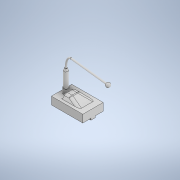
# Autodesk Inventor part: 準確無線麥克風組
Saved by Autodesk Inventor 2021 (Build 250183000, 183)
## iProperties
Created: 2023-02-28
Part Number: 準確無線麥克風組
Material: 一般
Document SubType Name: Modeling
Designer: brian
Density: 1 g/cm^3
Appearance: 預設
Author: brian
Autodesk Inventor part; units mm, degrees
ref_plane "YZ Plane" through (0, 0, 0) normal (1, 0, 0) x (0, 1, 0)
ref_plane "XZ Plane" through (0, 0, 0) normal (0, 1, 0) x (-1, 0, 0)
sketch "草圖1" plane through (0, 0, 0) normal (0, 1, 0) x (-1, 0, 0)
  line L0 (76.2, 49.6) -> (-76.2, 49.6)
  line L1 (-76.2, 49.6) -> (-76.2, -49.6)
  line L2 (-76.2, -49.6) -> (76.2, -49.6)
  line L3 (76.2, -49.6) -> (76.2, 49.6)
  line L4 (76.2, 49.6) -> (-76.2, -49.6) construction
  line L5 (-76.2, 49.6) -> (76.2, -49.6) construction
  point P0 (0, 0)
  dimension "d0" = 152.4
  dimension "d1" = 99.2
  constraints: 12 end point, 2 midpoint, 2 parallel, 1 horizontal, 1 perpendicular
  measures "d0" distance of L2.end L1.end
  measures "d1" distance of L1.end L0.end
extrude "擠出1" add sketch "草圖1" along normal blind 37
sketch "草圖2" plane through (0, 0, 0) normal (0, -1, 0) x (1, 0, 0)
  line L0 (76.2, 49.6) -> (76.2, -49.6) projected
  line L1 (65.2, 10) -> (76.2, 10)
  line L2 (76.2, 10) -> (76.2, -10)
  line L3 (76.2, -10) -> (65.2, -10)
  line L4 (65.2, -10) -> (65.2, 10)
  point P0 (0, 0)
  point P1 (65.2, 0)
  point P2 (76.2, 0)
  dimension "d4" = 20
  dimension "d5" = 11
  constraints: 8 end point, 2 midpoint, 2 parallel, 1 horizontal, 1 horizontal alignment, 1 perpendicular, 1 point on line
  measures "d4" distance of L3.end L1.start
  measures "d5" distance between parallel lines of L0 L4
extrude "擠出2" add sketch "草圖2" along normal blind 8
sketch "草圖3" plane through (0, 37, 0) normal (0, 1, 0) x (1, 0, 0)
  line L0 (-42.2, -36) -> (47.8, -36)
  line L1 (47.8, -36) -> (47.8, 36)
  line L2 (47.8, 36) -> (-42.2, 36)
  line L3 (-42.2, 36) -> (-42.2, -36)
  line L4 (-42.2, -36) -> (47.8, 36) construction
  line L5 (47.8, -36) -> (-42.2, 36) construction
  line L6 (-76.2, 49.6) -> (-76.2, -49.6) projected
  point P0 (2.8, 0)
  dimension "d8" = 90
  dimension "d9" = 72
  dimension "d14" = 34
  constraints: 12 end point, 2 midpoint, 2 parallel, 1 horizontal, 1 perpendicular
  measures "d8" distance of L2.end L1.end
  measures "d9" distance of L1.end L0.end
  measures "d14" distance between parallel lines of L6 L3
extrude "擠出3" add sketch "草圖3" along normal blind 16
sketch "草圖4" plane through (0, 37, 0) normal (0, 1, 0) x (1, 0, 0)
  circle A0 centre (-55.2, 0) radius 12.5
  line L0 (-76.2, 49.6) -> (-76.2, -49.6) projected
  point P0 (0, 0)
  point P1 (-76.2, 0)
  dimension "d12" = 25
  dimension "d13" = 21
  constraints: 1 centre point, 1 horizontal alignment, 1 midpoint
  measures "d12" diameter of A0
  measures "d13" distance from line of L0 A0.centre
extrude "擠出4" add sketch "草圖4" along normal blind 22
sketch "草圖5" plane through (-55.2, 59, 0) normal (0, 1, 0) x (1, 0, 0)
  circle A0 centre (0, 0) radius 12.5 projected
  circle A1 centre (0, 0) radius 10
  point P0 (55.2, 0)
  dimension "d17" = 20
  constraints: 1 centre point, 1 coincident
  measures "d17" diameter of A1
extrude "擠出5" add sketch "草圖5" along normal blind 72 contours A1
ref_plane "工作平面1" through (-55.2, 141, 0) normal (0, 1, 0) x (1, 0, 0)
sketch "草圖6" plane through (-55.2, 141, 0) normal (0, 1, 0) x (1, 0, 0)
  circle A0 centre (0, 0) radius 10 construction
  circle A1 centre (0, 0) radius 6.25
  point P0 (55.2, 0)
  dimension "d21" = 12.5
  constraints: 1 centre point, 1 coincident
  measures "d21" diameter of A1
loft "斷面混成1" add profiles "草圖6" section 1 edges at (-65.2, 131, 0)
sketch "草圖7" plane through (-55.2, 141, 0) normal (0, 1, 0) x (1, 0, 0)
  circle A0 centre (0, 0) radius 6.25 projected
  line L0 (0, 0) -> (147.496, -68.7785)
  line L1 (0, 0) -> (162.7438, 0) construction
  point P0 (55.2, 0)
  dimension "d26" = 25
  constraints: 4 end point, 1 equal length, 1 horizontal
  measures "d26" angle of L0 L1
surface extrude "擠出表面1" sketch "草圖7" along normal blind 72 shown no curves L0
sketch "草圖8" plane through (-55.2, 141, 0) normal (0.4226183, 0, -0.9063078) x (-0.9063078, 0, -0.4226183)
  line L0 (-6.25, 0) -> (6.25, 0) projected
  arc A0 (0, 0) -> (-52.6384, 75.1754) centre (-80, 0) ccw
  line L1 (-52.6384, 75.1754) -> (-406.9129, 204.1208)
  line L2 (12.5, -82) -> (-12.5, -82) projected
  point P0 (-50.0282, -141)
  dimension "d29" = 80
  dimension "d30" = 82
  dimension "d31" = 377.0111
  dimension "d32" = 70
  constraints: 2 end point, 2 point on circle, 1 centre point, 1 line through centre, 1 midpoint, 1 tangent
  measures "d29" radius of A0
  measures "d30" distance between parallel lines of L2 L0
  measures "d31" distance of L1.start L1.end
sketch "草圖9" plane through (-55.2, 141, 0) normal (0, 1, 0) x (1, 0, 0)
  circle A0 centre (0, 0) radius 6.25 projected
  circle A1 centre (0, 0) radius 4
  point P0 (55.2, 0)
  dimension "d33" = 8
  constraints: 1 centre point, 1 coincident
  measures "d33" diameter of A1
sweep "掃掠1" add profiles "草圖9" path "草圖8" path curves A0 L1 contours A1
sketch "草圖10" plane through (-55.2, 141, 0) normal (0.4226183, 0, -0.9063078) x (-0.9063078, 0, -0.4226183)
  line L0 (-405.5449, 207.8796) -> (-408.281, 200.362) projected
  arc A0 (-427.5295, 200.9828) -> (-408.281, 200.362) centre (-416.9585, 230.0264) ccw
  arc A1 (-405.5449, 207.8796) -> (-420.6891, 219.7767) centre (-431.2601, 190.7331) ccw
  arc A2 (-420.6891, 219.7767) -> (-427.5295, 200.9828) centre (-424.1093, 210.3798) ccw
  line L1 (-51.2703, 78.9342) -> (-405.5449, 207.8796) projected
  line L2 (-54.0065, 71.4166) -> (-408.281, 200.362) projected
  line L3 (-416.9585, 230.0264) -> (-431.2601, 190.7331) construction
  line L4 (-424.1093, 210.3798) -> (-406.9129, 204.1208) construction
  line L5 (-433.5062, 213.8) -> (-406.9129, 204.1208)
  point P0 (-50.0282, -141)
  dimension "d36" = 10
  dimension "d37" = 28.3
  constraints: 7 point on circle, 6 end point, 3 centre point, 2 midpoint, 2 perpendicular, 2 tangent, 1 coincident, 1 equal radius
  measures "d36" radius of A2
  measures "d37" distance from line of L0 L5.start
revolve "迴轉1" add sketch "草圖10" angle 360 about axis through (337.6901, 354.8, 183.2077) along (-0.8516507, -0.3420201, -0.3971313) contours L0 A0 A2 L5
chamfer "倒角1" distance 16 angle 45 2 edges at (2.8, 53, 36) (2.8, 53, -36)
chamfer "倒角2" distance 16 angle 75 1 edges at (47.8, 53, 0) measured on face at (47.8, 52.5, 0)
fillet "圓角1" radius 20 7 edges at (17.9436, 45.0001, 28) (47.8, 37.0001, 36) (17.9436, 45, -28.0001) (47.8, 37.0001, -36) (-27.0564, 53, 20.0001) (-11.9127, 53, 0) (-27.0564, 53, -20.0001)
fillet "圓角1" radius 5.25 5 edges at (-42.2, 53, 0) (-42.2, 45.0001, 28) (-42.2, 37.0001, 36) (-42.2, 37.0001, -36) (-42.2, 45.0001, -28.0001)
sketch "草圖12" plane through (0, 0, 0) normal (0, -1, 0) x (1, 0, 0)
  line L0 (65.2, 10) -> (76.2, 10) projected
  line L1 (76.2, 49.6) -> (76.2, 10) projected
  line L2 (-76.2, 49.6) -> (76.2, 49.6) projected
  line L3 (-76.2, -49.6) -> (-76.2, 49.6) projected
  line L4 (76.2, -49.6) -> (-76.2, -49.6) projected
  line L5 (76.2, -10) -> (76.2, -49.6) projected
  line L6 (76.2, -10) -> (65.2, -10) projected
  line L7 (65.2, -10) -> (65.2, 10) projected
  line L8 (-73.7, 47.1) -> (73.7, 47.1)
  line L9 (73.7, 47.1) -> (73.7, 12.5)
  line L10 (73.7, 12.5) -> (62.7, 12.5)
  line L11 (62.7, 12.5) -> (62.7, -12.5)
  line L12 (62.7, -12.5) -> (73.7, -12.5)
  line L13 (73.7, -12.5) -> (73.7, -47.1)
  line L14 (73.7, -47.1) -> (-73.7, -47.1)
  line L15 (-73.7, -47.1) -> (-73.7, 47.1)
  point P0 (0, 0)
  dimension "d56" = 2.5
  constraints: 16 end point, 7 other
  measures "d56" distance between parallel lines of L3 L15
extrude "擠出6" cut sketch "草圖12" against normal blind 25 contours L8 L9 L10 L11 L12 L13 L14 L15
sketch "草圖11" plane through (0, 0, 0) normal (0, -1, 0) x (1, 0, 0)
  line L0 (-76.2, -49.6) -> (-76.2, 49.6) projected
  line L1 (-12.2, -37.25) -> (-12.2, 37.25) construction
  circle A0 centre (-12.2, -37.25) radius 2.5
  circle A1 centre (-12.2, 37.25) radius 2.5
  circle A2 centre (-12.2, -37.25) radius 1.1
  circle A3 centre (-12.2, 37.25) radius 1.1
  point P0 (0, 0)
  point P1 (-12.2, 0)
  dimension "d47" = 74.5
  dimension "d48" = 64
  dimension "d59" = 5
  dimension "d60" = 5
  dimension "d61" = 2.2
  dimension "d62" = 2.2
  constraints: 4 centre point, 4 coincident, 2 end point, 1 horizontal alignment, 1 midpoint, 1 vertical, 1 vertical alignment
  measures "d47" distance of L1.end L1.start
  measures "d48" distance from line of L0 L1.start
  measures "d59" diameter of A0
  measures "d60" diameter of A1
  measures "d61" diameter of A2
  measures "d62" diameter of A3
extrude "擠出7" add sketch "草圖11" along normal blind 13.5 from surface at -25
equation "\"d60\" = d59"
equation "\"d62\" = d61"
equation "\"length\" = 585"
body "Srf1"
